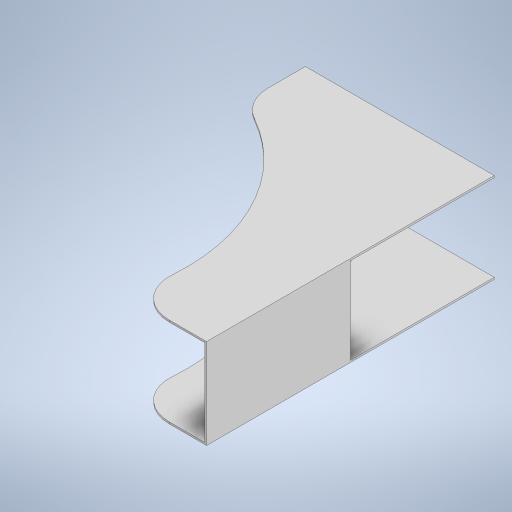
# Autodesk Inventor part: Soporte mangas
Saved by Autodesk Inventor 2023 (Build 270158000, 158)
## iProperties
Created: 2023-04-12
Part Number: Soporte mangas
Material: Genérico
Document SubType Name: Modeling
Designer: sergi
Density: 1 g/cm^3
Appearance: Valor por defecto
Author: sergi
Autodesk Inventor part; units mm, degrees
ref_plane "YZ Plane" through (0, 0, 0) normal (1, 0, 0) x (0, 1, 0)
ref_plane "XZ Plane" through (0, 0, 0) normal (0, 1, 0) x (-1, 0, 0)
ref_plane "XY Plane" through (0, 0, 0) normal (0, 0, 1) x (1, 0, 0)
sketch "Boceto1" plane through (0, 0, 0) normal (0, 1, 0) x (-1, 0, 0)
  line L0 (0, 0) -> (151, 0)
  line L1 (151, 0) -> (151, -230)
  line L2 (151, -230) -> (0, -230)
  line L3 (0, -230) -> (0, 0)
  dimension "d0" = 151
  dimension "d1" = 230
  constraints: 8 end point, 2 parallel, 1 horizontal, 1 perpendicular
  measures "d0" distance of L1.end L2.end
  measures "d1" distance of L0.end L1.end
extrude "Extrusión1" add sketch "Boceto1" along normal blind 72
shell "Vaciado1" thickness 1.5 removed faces 2 at (-151, 24, -153.3333) at (-100.6667, 24, 0)
sketch "Boceto2" plane through (0, 72, 0) normal (0, 1, 0) x (1, 0, 0)
  line L0 (-151, 0) -> (0, 0) projected
  line L1 (0, 0) -> (0, 230) projected
  circle A0 centre (-30, 30) radius 30
  circle A1 centre (-121, 200) radius 30
  line L2 (-151, 230) -> (-151, 0) projected
  line L3 (0, 230) -> (-151, 230) projected
  circle A2 centre (-209.5106, 43.2649) radius 150
  point P0 (-30, 0)
  point P1 (-59.9184, 32.2108)
  point P2 (-135.7518, 173.8775)
  point P3 (-151, 200)
  dimension "d5" = 60
  dimension "d6" = 60
  dimension "d7" = 300
  constraints: 6 tangent, 3 centre point
  measures "d5" diameter of A0
  measures "d6" diameter of A1
  measures "d7" diameter of A2
extrude "Extrusión2" cut sketch "Boceto2" against normal through all contours L2 A2 L0 | A2 A0 L0 | L2 A1 A2 picked at (-136.3795, 113.0822)
sketch "Boceto3" plane through (-1.5, 1.5, 0) normal (-1, 0, 0) x (0, 0, 1)
  line L0 (0, 0) -> (-228.5, 0) projected
  line L1 (0, 69) -> (0, 0) projected
  line L2 (0, 69) -> (-228.5, 69) projected
  line L3 (-228.5, 0) -> (-228.5, 69) projected
  line L4 (-228.5, 0) -> (-113.5, 0)
  line L5 (-113.5, 0) -> (-113.5, 69)
  line L6 (-113.5, 69) -> (-228.5, 69)
  line L7 (-228.5, 69) -> (-228.5, 0)
  point P0 (0, -1.5)
  dimension "d10" = 115
  constraints: 8 end point, 2 parallel, 1 horizontal, 1 perpendicular, 1 point on line
  measures "d10" distance of L6.end L5.end
extrude "Extrusión3" add sketch "Boceto3" along normal blind 75.5 contours L0 L3 L2 L5
shell "Vaciado2" thickness 1.5 removed faces 2 at (0, 24, -76.6667) at (-50.3333, 24, -230)
fillet "Empalme1" radius 115 3 edges at (-75.5, 2.25, -115) (-75.5, 36, -115) (-75.5, 69.75, -115)
